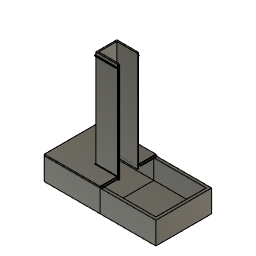
Tower+Base (Autodesk Fusion 360 design; units mm, degrees)
Autodesk Fusion 360 part; units mm, degrees
(part 1 of 2)
sketch "Sketch1" plane through (0, 0, 0) normal (0, 0, 1) x (1, 0, 0)
  line L0 (-38.1, 25.4) -> (469.9, 25.4)
  line L1 (469.9, 25.4) -> (469.9, -482.6)
  line L2 (469.9, -482.6) -> (-38.1, -482.6)
  line L3 (-38.1, -482.6) -> (-38.1, 25.4)
  dimension "d9" = 508
  dimension "d10" = 508
  constraint horizontal L0
  constraint vertical L1
  constraint horizontal L2
  constraint vertical L3
  measures "d9" distance of L0.start L0.end
  measures "d10" distance of L0.start L2.end
extrude "Extrude1" add sketch "Sketch1" along normal blind 203.2 makes body 1
sketch "Sketch2" plane through (0, 0, 203.2) normal (0, 0, 1) x (-1, 0, 0)
  line L0 (38.1, 482.6) -> (-469.9, 482.6)
  line L1 (-469.9, 482.6) -> (-469.9, -25.4)
  line L2 (-469.9, -25.4) -> (38.1, -25.4)
  line L3 (38.1, -25.4) -> (38.1, 482.6)
  line L4 (-469.9, 0) -> (12.7, 0)
  line L5 (12.7, 0) -> (12.7, 457.2)
  line L6 (12.7, 457.2) -> (-469.9, 457.2)
  line L7 (-469.9, 457.2) -> (-469.9, 0)
  dimension "d13" = 25.4
  dimension "d14" = 25.4
  dimension "d15" = 25.4
  constraint horizontal L4
  constraint vertical L5
  constraint horizontal L6
  constraint vertical L7
  constraint coincident L1 L4.start
  measures "d13" distance of L2 L4
  measures "d14" distance of L3 L5
  measures "d15" distance of L0 L6
extrude "Extrude2" cut sketch "Sketch2" against normal blind 177.8 contours L1 L4 L5 L6 L7 bodies 1
sketch "Sketch3" plane through (469.9, 0, 0) normal (1, 0, 0) x (0, 1, 0)
  line L0 (0, 203.2) -> (0, 25.4)
  line L1 (0, 25.4) -> (-457.2, 25.4)
  line L2 (-457.2, 25.4) -> (-457.2, 203.2)
  line L3 (-457.2, 203.2) -> (-482.6, 203.2)
  line L4 (-482.6, 203.2) -> (-482.6, 0)
  line L5 (-482.6, 0) -> (25.4, 0)
  line L6 (25.4, 0) -> (25.4, 203.2)
  line L7 (25.4, 203.2) -> (0, 203.2)
  line L8 (-457.2, 203.2) -> (-469.9, 203.2)
  line L9 (-469.9, 203.2) -> (-469.9, 12.7)
  line L10 (-469.9, 12.7) -> (-101.6, 12.7)
  line L11 (-101.6, 12.7) -> (12.7, 12.7)
  line L12 (12.7, 12.7) -> (12.7, 25.4)
  line L13 (0, 203.2) -> (12.7, 203.2)
  line L14 (12.7, 203.2) -> (12.7, 25.4)
  line L15 (0, 25.4) -> (0, 203.2)
  dimension "d20" = 12.7
  dimension "d21" = 12.7
  dimension "d22" = 12.7
  constraint horizontal L8
  constraint vertical L9
  constraint horizontal L10
  constraint coincident L2.end L3.start
  constraint horizontal L11
  constraint vertical L12
  constraint horizontal L13
  constraint vertical L14
  constraint vertical L15
  constraint coincident L0.start L7.end
  measures "d20" distance of L4 L9
  measures "d21" distance of L5 L11
  measures "d22" distance of L6 L14
extrude "Extrude3" add sketch "Sketch3" along normal blind 6.35 contours L0 L1 L2 L3 L7 L8 L9 L10 L11 L12 L13 L14 L15 bodies 1
move_body "Move1" bodies 1 to x (1, 0, 0) y (0, 1, 0) z (0, 0, 1) at (-317.5, 0, 0)
sketch "Sketch4" plane through (0, 0, 0) normal (0, 0, 1) x (1, 0, 0)
  line L0 (-127, 25.4) -> (381, 25.4)
  line L1 (381, 25.4) -> (381, -482.6)
  line L2 (381, -482.6) -> (-127, -482.6)
  line L3 (-127, -482.6) -> (-127, 25.4)
  dimension "d26" = 508
  dimension "d27" = 508
  constraint horizontal L0
  constraint vertical L1
  constraint horizontal L2
  constraint vertical L3
  measures "d26" distance of L0.start L0.end
  measures "d27" distance of L0.end L1.end
extrude "Extrude4" add sketch "Sketch4" along normal blind 203.2 separate body makes body 2
sketch "Sketch5" plane through (0, 0, 203.2) normal (0, 0, 1) x (-1, 0, 0)
  line L0 (127, 482.6) -> (-381, 482.6)
  line L1 (-381, 482.6) -> (-381, -25.4)
  line L2 (-381, -25.4) -> (127, -25.4)
  line L3 (127, -25.4) -> (127, 482.6)
  line L4 (127, 0) -> (-355.6, 0)
  line L5 (-355.6, 0) -> (-355.6, 457.2)
  line L6 (-355.6, 457.2) -> (127, 457.2)
  line L7 (127, 457.2) -> (127, 0)
  dimension "d30" = 25.4
  dimension "d31" = 25.4
  dimension "d32" = 25.4
  constraint horizontal L4
  constraint vertical L5
  constraint horizontal L6
  constraint vertical L7
  constraint coincident L3 L4.start
  measures "d30" distance of L2 L4
  measures "d31" distance of L1 L5
  measures "d32" distance of L0 L6
extrude "Extrude5" cut sketch "Sketch5" against normal blind 177.8 contours L3 L4 L5 L6 L7 bodies 2
sketch "Sketch6" plane through (-127, 0, 0) normal (-1, 0, 0) x (0, -1, 0)
  line L0 (457.2, 203.2) -> (457.2, 25.4)
  line L1 (457.2, 25.4) -> (0, 25.4)
  line L2 (0, 25.4) -> (0, 203.2)
  line L3 (0, 203.2) -> (-25.4, 203.2)
  line L4 (-25.4, 203.2) -> (-25.4, 0)
  line L5 (-25.4, 0) -> (482.6, 0)
  line L6 (482.6, 0) -> (482.6, 203.2)
  line L7 (482.6, 203.2) -> (457.2, 203.2)
  line L8 (0, 203.2) -> (-12.7, 203.2)
  line L9 (-12.7, 203.2) -> (-12.7, 12.7)
  line L10 (-12.7, 12.7) -> (0, 12.7)
  line L11 (0, 12.7) -> (469.9, 12.7)
  line L12 (469.9, 12.7) -> (469.9, 25.4)
  line L13 (457.2, 25.4) -> (457.2, 203.2)
  line L14 (457.2, 203.2) -> (469.9, 203.2)
  line L15 (469.9, 203.2) -> (469.9, 25.4)
  dimension "d35" = 12.7
  dimension "d36" = 12.7
  dimension "d37" = 12.7
  constraint horizontal L8
  constraint vertical L9
  constraint horizontal L10
  constraint coincident L2.end L3.start
  constraint horizontal L11
  constraint vertical L12
  constraint vertical L13
  constraint horizontal L14
  constraint vertical L15
  constraint coincident L0.start L7.end
  measures "d35" distance of L2 L9
  measures "d36" distance of L13 L15
  measures "d37" distance of L1 L11
extrude "Extrude6" cut sketch "Sketch6" against normal blind 6.35 contours L0 L1 L2 L3 L7 L8 L9 L10 L11 L12 L13 L14 L15 bodies 2
sketch "Sketch7" plane through (0, 0, 0) normal (0, 0, 1) x (1, 0, 0)
  line L0 (-457.2, 177.8) -> (50.8, 177.8)
  line L1 (50.8, 177.8) -> (50.8, -330.2)
  line L2 (50.8, -330.2) -> (-457.2, -330.2)
  line L3 (-457.2, -330.2) -> (-457.2, 177.8)
  line L4 (50.8, 25.4) -> (-152.4, 25.4)
  line L5 (-152.4, 25.4) -> (-152.4, -177.8)
  line L6 (-152.4, -177.8) -> (50.8, -177.8)
  line L7 (50.8, -177.8) -> (50.8, 25.4)
  dimension "d40" = 508
  dimension "d41" = 508
  dimension "d42" = 203.2
  dimension "d43" = 203.2
  dimension "d87" = 152.4
  constraint horizontal L0
  constraint vertical L1
  constraint horizontal L2
  constraint vertical L3
  constraint horizontal L4
  constraint vertical L5
  constraint horizontal L6
  constraint vertical L7
  constraint coincident L1 L4.start
  measures "d40" distance of L0.start L0.end
  measures "d41" distance of L0.start L2.end
  measures "d42" distance of L4.end L5.end
  measures "d43" distance of L4.start L4.end
  measures "d87" distance of L0 L4
extrude "Extrude7" add sketch "Sketch7" along normal blind 12.7 separate body contours L0 L1 L2 L3 L4 L5 L6 makes body 3
sketch "Sketch8" plane through (50.8, 0, 0) normal (1, 0, 0) x (0, 1, 0)
  line L0 (-330.2, 0) -> (-177.8, 0)
  line L1 (-177.8, 0) -> (-177.8, 12.7)
  line L2 (-177.8, 12.7) -> (-330.2, 12.7)
  line L3 (-330.2, 12.7) -> (-330.2, 0)
  line L4 (-330.2, 6.35) -> (-177.8, 6.35)
  line L5 (-177.8, 6.35) -> (-177.8, 0)
  line L6 (-177.8, 0) -> (-330.2, 0)
  line L7 (-330.2, 0) -> (-330.2, 6.35)
  dimension "d47" = 6.35
  constraint horizontal L4
  constraint vertical L5
  constraint horizontal L6
  constraint vertical L7
  constraint coincident L0.end L1.start
  constraint coincident L3 L4.start
  measures "d47" distance of L4.start L0.start
extrude "Extrude8" add sketch "Sketch8" along normal blind 12.7 contours L0 L1 L3 L4 L5 L6 L7 bodies 3
sketch "Sketch9" plane through (-152.4, 0, 0) normal (1, 0, 0) x (0, 1, 0)
  line L0 (-177.8, 0) -> (25.4, 0)
  line L1 (25.4, 0) -> (25.4, 12.7)
  line L2 (25.4, 12.7) -> (-177.8, 12.7)
  line L3 (-177.8, 12.7) -> (-177.8, 0)
  line L4 (-177.8, 0) -> (25.4, 0)
  line L5 (25.4, 0) -> (25.4, 6.35)
  line L6 (25.4, 6.35) -> (-177.8, 6.35)
  line L7 (-177.8, 6.35) -> (-177.8, 0)
  dimension "d51" = 6.35
  constraint horizontal L4
  constraint vertical L5
  constraint horizontal L6
  constraint vertical L7
  constraint coincident L1 L5.end
  constraint coincident L0.start L3.end
  measures "d51" distance of L0.start L6.end
extrude "Extrude9" add sketch "Sketch9" along normal blind 12.7 contours L0 L1 L3 L4 L5 L6 L7 bodies 3
sketch "Sketch10" plane through (50.8, 0, 0) normal (1, 0, 0) x (0, 1, 0)
  line L0 (25.4, 0) -> (177.8, 0)
  line L1 (177.8, 0) -> (177.8, 12.7)
  line L2 (177.8, 12.7) -> (25.4, 12.7)
  line L3 (25.4, 12.7) -> (25.4, 0)
  line L4 (25.4, 0) -> (177.8, 0)
  line L5 (177.8, 0) -> (177.8, 6.35)
  line L6 (177.8, 6.35) -> (25.4, 6.35)
  line L7 (25.4, 6.35) -> (25.4, 0)
  dimension "d54" = 6.35
  constraint horizontal L4
  constraint vertical L5
  constraint horizontal L6
  constraint vertical L7
  constraint coincident L1 L5.end
  constraint coincident L0.start L3.end
  measures "d54" distance of L0.start L6.end
extrude "Extrude10" add sketch "Sketch10" along normal blind 12.7 contours L0 L1 L3 L4 L5 L6 L7 bodies 3
sketch "Sketch11" plane through (0, -177.8, 0) normal (0, 1, 0) x (-1, 0, 0)
  line L0 (139.7, 6.35) -> (152.4, 6.35)
  line L1 (152.4, 6.35) -> (152.4, 12.7)
  line L2 (152.4, 12.7) -> (-50.8, 12.7)
  line L3 (-50.8, 12.7) -> (-50.8, 6.35)
  line L4 (-50.8, 6.35) -> (-63.5, 6.35)
  line L5 (-63.5, 6.35) -> (-63.5, 0)
  line L6 (-63.5, 0) -> (139.7, 0)
  line L7 (139.7, 0) -> (139.7, 6.35)
  line L8 (-50.8, 6.35) -> (139.7, 6.35)
  line L9 (139.7, 6.35) -> (139.7, 0)
  line L10 (139.7, 0) -> (-50.8, 0)
  line L11 (-50.8, 0) -> (-50.8, 6.35)
  constraint horizontal L8
  constraint vertical L9
  constraint horizontal L10
  constraint vertical L11
  constraint coincident L6.end L7.start
  constraint coincident L3.end L4.start
extrude "Extrude11" add sketch "Sketch11" along normal blind 12.7 contours L6 L7 L8 L9 L10 L11 bodies 3
sketch "Sketch12" plane through (0, 25.4, 0) normal (0, -1, 0) x (1, 0, 0)
  line L0 (-152.4, 6.35) -> (-139.7, 6.35)
  line L1 (-139.7, 6.35) -> (-139.7, 0)
  line L2 (-139.7, 0) -> (63.5, 0)
  line L3 (63.5, 0) -> (63.5, 6.35)
  line L4 (63.5, 6.35) -> (50.8, 6.35)
  line L5 (50.8, 6.35) -> (50.8, 12.7)
  line L6 (50.8, 12.7) -> (-152.4, 12.7)
  line L7 (-152.4, 12.7) -> (-152.4, 6.35)
  line L8 (-139.7, 0) -> (50.8, 0)
  line L9 (50.8, 0) -> (50.8, 6.35)
  line L10 (50.8, 6.35) -> (-139.7, 6.35)
  line L11 (-139.7, 6.35) -> (-139.7, 0)
  constraint horizontal L8
  constraint vertical L9
  constraint horizontal L10
  constraint vertical L11
  constraint coincident L4.end L5.start
  constraint coincident L1.end L2.start
extrude "Extrude12" add sketch "Sketch12" along normal blind 12.7 contours L1 L2 L8 L9 L10 L11 bodies 3
sketch "Sketch13" plane through (0, 0, 0) normal (0, 0, 1) x (1, 0, 0)
  line L0 (-152.4, 177.8) -> (355.6, 177.8)
  line L1 (355.6, 177.8) -> (355.6, -330.2)
  line L2 (355.6, -330.2) -> (-152.4, -330.2)
  line L3 (-152.4, -330.2) -> (-152.4, 177.8)
  line L4 (-152.4, 25.4) -> (50.8, 25.4)
  line L5 (50.8, 25.4) -> (50.8, -177.8)
  line L6 (50.8, -177.8) -> (-152.4, -177.8)
  line L7 (-152.4, -177.8) -> (-152.4, 25.4)
  dimension "d61" = 508
  dimension "d62" = 508
  dimension "d63" = 203.2
  dimension "d64" = 203.2
  dimension "d88" = 152.4
  constraint horizontal L0
  constraint vertical L1
  constraint horizontal L2
  constraint vertical L3
  constraint horizontal L4
  constraint vertical L5
  constraint horizontal L6
  constraint vertical L7
  constraint coincident L3 L4.start
  measures "d61" distance of L0.start L0.end
  measures "d62" distance of L0.end L1.end
  measures "d63" distance of L4.start L4.end
  measures "d64" distance of L4.end L5.end
  measures "d88" distance of L0 L4
extrude "Extrude13" add sketch "Sketch13" along normal blind 12.7 separate body contours L0 L1 L2 L3 L4 L5 L6 makes body 4
sketch "Sketch14" plane through (-152.4, 0, 0) normal (-1, 0, 0) x (0, -1, 0)
  line L0 (-177.8, 0) -> (-25.4, 0)
  line L1 (-25.4, 0) -> (-25.4, 12.7)
  line L2 (-25.4, 12.7) -> (-177.8, 12.7)
  line L3 (-177.8, 12.7) -> (-177.8, 0)
  line L4 (-177.8, 0) -> (-25.4, 0)
  line L5 (-25.4, 0) -> (-25.4, 6.35)
  line L6 (-25.4, 6.35) -> (-177.8, 6.35)
  line L7 (-177.8, 6.35) -> (-177.8, 0)
  dimension "d67" = 6.35
  constraint horizontal L4
  constraint vertical L5
  constraint horizontal L6
  constraint vertical L7
  constraint coincident L1 L5.end
  constraint coincident L0.start L3.end
  measures "d67" distance of L0.start L6.end
extrude "Extrude14" cut sketch "Sketch14" against normal blind 12.7 contours L0 L1 L3 L4 L5 L6 L7 bodies 4
sketch "Sketch15" plane through (-152.4, 0, 0) normal (-1, 0, 0) x (0, -1, 0)
  line L0 (177.8, 0) -> (330.2, 0)
  line L1 (330.2, 0) -> (330.2, 12.7)
  line L2 (330.2, 12.7) -> (177.8, 12.7)
  line L3 (177.8, 12.7) -> (177.8, 0)
  line L4 (177.8, 0) -> (330.2, 0)
  line L5 (330.2, 0) -> (330.2, 6.35)
  line L6 (330.2, 6.35) -> (177.8, 6.35)
  line L7 (177.8, 6.35) -> (177.8, 0)
  dimension "d70" = 6.35
  constraint horizontal L4
  constraint vertical L5
  constraint horizontal L6
  constraint vertical L7
  constraint coincident L1 L5.end
  constraint coincident L0.start L3.end
  measures "d70" distance of L0.start L6.end
extrude "Extrude15" cut sketch "Sketch15" against normal blind 12.7 contours L0 L1 L3 L4 L5 L6 L7 bodies 4
sketch "Sketch16" plane through (50.8, 0, 0) normal (-1, 0, 0) x (0, -1, 0)
  line L0 (-25.4, 0) -> (177.8, 0)
  line L1 (177.8, 0) -> (177.8, 12.7)
  line L2 (177.8, 12.7) -> (-25.4, 12.7)
  line L3 (-25.4, 12.7) -> (-25.4, 0)
  line L4 (-25.4, 0) -> (177.8, 0)
  line L5 (177.8, 0) -> (177.8, 12.7)
  line L6 (177.8, 12.7) -> (-25.4, 12.7)
  line L7 (-25.4, 12.7) -> (-25.4, 0)
  dimension "d73" = 12.7
  constraint horizontal L4
  constraint vertical L5
  constraint horizontal L6
  constraint vertical L7
  constraint coincident L1 L2.start
  constraint coincident L0.start L3.end
  measures "d73" distance of L0.start L2.end
extrude "Extrude16" add sketch "Sketch16" along normal blind 12.7 bodies 4
sketch "Sketch17" plane through (0, 25.4, 0) normal (0, -1, 0) x (1, 0, 0)
  line L0 (38.1, 0) -> (38.1, 12.7)
  line L1 (-152.4, 12.7) -> (-152.4, 6.35)
  line L2 (-152.4, 6.35) -> (-139.7, 6.35)
  line L3 (-139.7, 6.35) -> (-139.7, 0)
  line L4 (-139.7, 0) -> (38.1, 0)
  line L5 (-139.7, 0) -> (38.1, 0)
  line L6 (38.1, 0) -> (38.1, 12.7)
  line L7 (38.1, 12.7) -> (-139.7, 12.7)
  line L8 (-139.7, 12.7) -> (-139.7, 0)
  line L9 (38.1, 12.7) -> (-152.4, 12.7)
  constraint horizontal L5
  constraint vertical L6
  constraint horizontal L7
  constraint vertical L8
  constraint coincident L0.end L6.end
  constraint coincident L3.end L4.start
extrude "Extrude17" add sketch "Sketch17" along normal blind 12.7 contours L0 L3 L4 L5 L6 L7 L8 L9 bodies 4
sketch "Sketch18" plane through (0, -177.8, 0) normal (0, 1, 0) x (-1, 0, 0)
  line L0 (152.4, 12.7) -> (-38.1, 12.7)
  line L1 (-38.1, 12.7) -> (-38.1, 0)
  line L2 (-38.1, 0) -> (139.7, 0)
  line L3 (139.7, 0) -> (139.7, 6.35)
  line L4 (139.7, 6.35) -> (152.4, 6.35)
  line L5 (152.4, 6.35) -> (152.4, 12.7)
  line L6 (-38.1, 0) -> (139.7, 0)
  line L7 (139.7, 0) -> (139.7, 6.35)
  line L8 (139.7, 6.35) -> (-38.1, 6.35)
  line L9 (-38.1, 6.35) -> (-38.1, 0)
  constraint horizontal L6
  constraint vertical L7
  constraint horizontal L8
  constraint vertical L9
  constraint coincident L3.end L4.start
  constraint coincident L1.end L2.start
extrude "Extrude18" add sketch "Sketch18" along normal blind 12.7 contours L1 L2 L3 L6 L7 L8 L9 bodies 4
sketch "Sketch19" plane through (-139.7, 0, 0) normal (-1, 0, 0) x (0, -1, 0)
  line L0 (-177.8, 6.35) -> (-177.8, 0)
  line L1 (-177.8, 0) -> (-12.7, 0)
  line L2 (-12.7, 0) -> (-12.7, 12.7)
  line L3 (-12.7, 12.7) -> (-25.4, 12.7)
  line L4 (-25.4, 6.35) -> (-177.8, 6.35)
  line L5 (-25.4, 12.7) -> (-12.7, 12.7)
  line L6 (-12.7, 12.7) -> (-12.7, 0)
  line L7 (-12.7, 0) -> (-25.4, 0)
  line L8 (-25.4, 0) -> (-25.4, 12.7)
  line L9 (-25.4, 12.7) -> (-25.4, 6.35)
  constraint horizontal L5
  constraint vertical L6
  constraint horizontal L7
  constraint vertical L8
  constraint coincident L1.end L2.start
  constraint coincident L3.end L5.start
sketch "Sketch20" plane through (-139.7, 0, 0) normal (-1, 0, 0) x (0, -1, 0)
  line L0 (165.1, 0) -> (330.2, 0)
  line L1 (330.2, 0) -> (330.2, 6.35)
  line L2 (330.2, 6.35) -> (177.8, 6.35)
  line L3 (177.8, 6.35) -> (165.1, 6.35)
  line L4 (165.1, 6.35) -> (165.1, 0)
  line L5 (165.1, 6.35) -> (177.8, 6.35)
  line L6 (177.8, 6.35) -> (177.8, 0)
  line L7 (177.8, 0) -> (165.1, 0)
  line L8 (165.1, 0) -> (165.1, 6.35)
  constraint horizontal L5
  constraint vertical L6
  constraint horizontal L7
  constraint vertical L8
  constraint coincident L0 L6.end
  constraint coincident L3.end L4.start
extrude "Extrude20" add sketch "Sketch20" along normal blind 12.7 separate body contours L0 L3 L4 L5 L6 L7 L8 makes body 5
sketch "Sketch21" plane through (-139.7, 0, 0) normal (-1, 0, 0) x (0, -1, 0)
  line L0 (-177.8, 6.35) -> (-177.8, 0)
  line L1 (-177.8, 0) -> (-12.7, 0)
  line L2 (-12.7, 0) -> (-12.7, 12.7)
  line L3 (-12.7, 12.7) -> (-25.4, 12.7)
  line L4 (-25.4, 6.35) -> (-177.8, 6.35)
  line L5 (-25.4, 12.7) -> (-12.7, 12.7)
  line L6 (-12.7, 12.7) -> (-12.7, 0)
  line L7 (-12.7, 0) -> (-25.4, 0)
  line L8 (-25.4, 0) -> (-25.4, 12.7)
  line L9 (-25.4, 12.7) -> (-25.4, 6.35)
  constraint horizontal L5
  constraint vertical L6
  constraint horizontal L7
  constraint vertical L8
  constraint coincident L1.end L2.start
  constraint coincident L3.end L5.start
extrude "Extrude21" add sketch "Sketch21" along normal blind 12.7 separate body contours L1 L2 L3 L5 L6 L7 L8 L9 makes body 6
combine "Combine1" operation add target body 6 tool bodies 4 5
sketch "Sketch22" plane through (0, 0, 0) normal (0, 0, 1) x (1, 0, 0)
sketch "Sketch23" plane through (0, 0, 0) normal (0, 0, 1) x (1, 0, 0)
sketch "Sketch24" plane through (0, 314.0699, 0) normal (0, 1, 0) x (-1, 0, 0)
  line L0 (-261.6067, 0) -> (-198.1067, 0)
  line L1 (-198.1067, 0) -> (-198.1067, 152.4)
  line L2 (-198.1067, 152.4) -> (-261.6067, 152.4)
  line L3 (-261.6067, 152.4) -> (-261.6067, 0)
  line L4 (-261.6067, 25.4) -> (-198.1067, 25.4)
  line L5 (-198.1067, 25.4) -> (-198.1067, 38.1)
  line L6 (-198.1067, 38.1) -> (-261.6067, 38.1)
  line L7 (-261.6067, 38.1) -> (-261.6067, 25.4)
  dimension "d96" = 25.4
  dimension "d97" = 12.7
  constraint horizontal L4
  constraint vertical L5
  constraint horizontal L6
  constraint vertical L7
  constraint coincident L1 L5.end
  constraint coincident L3 L4.start
  measures "d96" distance of L0 L4
  measures "d97" distance of L4.start L6.end
sketch "Sketch25" plane through (0, 314.0699, 0) normal (0, 1, 0) x (-1, 0, 0)
  line L0 (-261.6067, 38.1) -> (-198.1067, 38.1)
  line L1 (-198.1067, 38.1) -> (-198.1067, 152.4)
  line L2 (-198.1067, 152.4) -> (-261.6067, 152.4)
  line L3 (-261.6067, 152.4) -> (-261.6067, 38.1)
  line L4 (-261.6067, 127) -> (-198.1067, 127)
  line L5 (-198.1067, 127) -> (-198.1067, 114.3)
  line L6 (-198.1067, 114.3) -> (-261.6067, 114.3)
  line L7 (-261.6067, 114.3) -> (-261.6067, 127)
  dimension "d100" = 25.4
  dimension "d101" = 12.7
  constraint horizontal L4
  constraint vertical L5
  constraint horizontal L6
  constraint vertical L7
  constraint coincident L1 L5.end
  constraint coincident L3 L4.start
  measures "d100" distance of L2 L4
  measures "d101" distance of L4.end L5.end
sketch "Sketch26" plane through (0, 187.0699, 0) normal (0, -1, 0) x (1, 0, 0)
  line L0 (198.1067, 0) -> (261.6067, 0)
  line L1 (261.6067, 0) -> (261.6067, 152.4)
  line L2 (261.6067, 152.4) -> (198.1067, 152.4)
  line L3 (198.1067, 152.4) -> (198.1067, 0)
  line L4 (198.1067, 127) -> (261.6067, 127)
  line L5 (261.6067, 127) -> (261.6067, 114.3)
  line L6 (261.6067, 114.3) -> (198.1067, 114.3)
  line L7 (198.1067, 114.3) -> (198.1067, 127)
  dimension "d104" = 12.7
  dimension "d105" = 25.4
  constraint horizontal L4
  constraint vertical L5
  constraint horizontal L6
  constraint vertical L7
  constraint coincident L1 L5.end
  constraint coincident L3 L4.start
  measures "d104" distance of L4.start L6.end
  measures "d105" distance of L2 L4
sketch "Sketch27" plane through (0, 187.0699, 0) normal (0, -1, 0) x (1, 0, 0)
  line L0 (261.6067, 114.3) -> (198.1067, 114.3)
  line L1 (198.1067, 114.3) -> (198.1067, 0)
  line L2 (198.1067, 0) -> (261.6067, 0)
  line L3 (261.6067, 0) -> (261.6067, 114.3)
  line L4 (198.1067, 25.4) -> (261.6067, 25.4)
  line L5 (261.6067, 25.4) -> (261.6067, 38.1)
  line L6 (261.6067, 38.1) -> (198.1067, 38.1)
  line L7 (198.1067, 38.1) -> (198.1067, 25.4)
  dimension "d108" = 25.4
  dimension "d109" = 12.7
  constraint horizontal L4
  constraint vertical L5
  constraint horizontal L6
  constraint vertical L7
  constraint coincident L3 L5.end
  constraint coincident L1 L4.start
  measures "d108" distance of L2 L4
  measures "d109" distance of L4 L6
sketch "Sketch28" plane through (198.1067, 0, 0) normal (-1, 0, 0) x (0, -1, 0)
  line L0 (-314.0699, 127) -> (-326.7699, 127)
  line L1 (-326.7699, 127) -> (-326.7699, 114.3)
  line L2 (-326.7699, 114.3) -> (-314.0699, 114.3)
  line L3 (-326.7699, 127) -> (-174.3699, 127)
  line L4 (-174.3699, 127) -> (-174.3699, 114.3)
  line L5 (-174.3699, 114.3) -> (-326.7699, 114.3)
  line L6 (-326.7699, 114.3) -> (-326.7699, 127)
  line L7 (-314.0699, 114.3) -> (-314.0699, 127)
  constraint horizontal L3
  constraint vertical L4
  constraint horizontal L5
  constraint vertical L6
  constraint coincident L0.end L1.start
sketch "Sketch29" plane through (198.1067, 0, 0) normal (-1, 0, 0) x (0, -1, 0)
  line L0 (-314.0699, 38.1) -> (-326.7699, 38.1)
  line L1 (-326.7699, 38.1) -> (-326.7699, 25.4)
  line L2 (-326.7699, 25.4) -> (-314.0699, 25.4)
  line L3 (-326.7699, 38.1) -> (-174.3699, 38.1)
  line L4 (-174.3699, 38.1) -> (-174.3699, 25.4)
  line L5 (-174.3699, 25.4) -> (-326.7699, 25.4)
  line L6 (-326.7699, 25.4) -> (-326.7699, 38.1)
  line L7 (-314.0699, 25.4) -> (-314.0699, 38.1)
  constraint horizontal L3
  constraint vertical L4
  constraint horizontal L5
  constraint vertical L6
  constraint coincident L0.end L1.start
sketch "Sketch30" plane through (299.7067, 0, 0) normal (-1, 0, 0) x (0, -1, 0)
  line L0 (-301.3699, 0) -> (-288.6699, 0)
  line L1 (-288.6699, 0) -> (-288.6699, 152.4)
  line L2 (-288.6699, 152.4) -> (-301.3699, 152.4)
  line L3 (-301.3699, 152.4) -> (-301.3699, 127)
  line L4 (-301.3699, 127) -> (-314.0699, 127)
  line L5 (-314.0699, 127) -> (-314.0699, 114.3)
  line L6 (-314.0699, 114.3) -> (-301.3699, 114.3)
  line L7 (-301.3699, 114.3) -> (-301.3699, 38.1)
  line L8 (-301.3699, 38.1) -> (-314.0699, 38.1)
  line L9 (-314.0699, 38.1) -> (-314.0699, 25.4)
  line L10 (-314.0699, 25.4) -> (-301.3699, 25.4)
  line L11 (-301.3699, 25.4) -> (-301.3699, 0)
  line L12 (-288.6699, 0) -> (-295.0199, 0)
  line L13 (-295.0199, 0) -> (-295.0199, 152.4)
  line L14 (-295.0199, 152.4) -> (-288.6699, 152.4)
  line L15 (-288.6699, 152.4) -> (-288.6699, 0)
  constraint horizontal L12
  constraint vertical L13
  constraint horizontal L14
  constraint vertical L15
  constraint midpoint L2 L13.end
  constraint coincident L0.end L1.start
sketch "Sketch31" plane through (287.0067, 0, 0) normal (-1, 0, 0) x (0, -1, 0)
  line L0 (-288.6699, 152.4) -> (-295.0199, 152.4)
  line L1 (-295.0199, 152.4) -> (-295.0199, 0)
  line L2 (-295.0199, 0) -> (-288.6699, 0)
  line L3 (-288.6699, 0) -> (-288.6699, 152.4)
  line L4 (-295.0199, 152.4) -> (-288.6699, 152.4)
  line L5 (-288.6699, 152.4) -> (-288.6699, 139.7)
  line L6 (-288.6699, 139.7) -> (-295.0199, 139.7)
  line L7 (-295.0199, 139.7) -> (-295.0199, 152.4)
  dimension "d120" = 12.7
  constraint horizontal L4
  constraint vertical L5
  constraint horizontal L6
  constraint vertical L7
  constraint coincident L3 L5.end
  constraint coincident L0.end L1.start
  measures "d120" distance of L0.end L6.end
sketch "Sketch32" plane through (299.7067, 0, 0) normal (-1, 0, 0) x (0, -1, 0)
  line L0 (-187.0699, 0) -> (-174.3699, 0)
  line L1 (-174.3699, 0) -> (-174.3699, 25.4)
  line L2 (-174.3699, 25.4) -> (-161.6699, 25.4)
  line L3 (-161.6699, 25.4) -> (-161.6699, 38.1)
  line L4 (-161.6699, 38.1) -> (-174.3699, 38.1)
  line L5 (-174.3699, 38.1) -> (-174.3699, 114.3)
  line L6 (-174.3699, 114.3) -> (-161.6699, 114.3)
  line L7 (-161.6699, 114.3) -> (-161.6699, 127)
  line L8 (-161.6699, 127) -> (-174.3699, 127)
  line L9 (-174.3699, 127) -> (-174.3699, 152.4)
  line L10 (-174.3699, 152.4) -> (-187.0699, 152.4)
  line L11 (-187.0699, 152.4) -> (-187.0699, 0)
  line L12 (-187.0699, 152.4) -> (-180.7199, 152.4)
  line L13 (-180.7199, 152.4) -> (-180.7199, 0)
  line L14 (-180.7199, 0) -> (-187.0699, 0)
  line L15 (-187.0699, 0) -> (-187.0699, 152.4)
  constraint horizontal L12
  constraint vertical L13
  constraint horizontal L14
  constraint vertical L15
  constraint midpoint L0 L13.end
  constraint coincident L10.end L11.start
sketch "Sketch33" plane through (287.0067, 0, 0) normal (-1, 0, 0) x (0, -1, 0)
  line L0 (-187.0699, 0) -> (-180.7199, 0)
  line L1 (-180.7199, 0) -> (-180.7199, 152.4)
  line L2 (-180.7199, 152.4) -> (-187.0699, 152.4)
  line L3 (-187.0699, 152.4) -> (-187.0699, 0)
  line L4 (-187.0699, 152.4) -> (-180.7199, 152.4)
  line L5 (-180.7199, 152.4) -> (-180.7199, 139.7)
  line L6 (-180.7199, 139.7) -> (-187.0699, 139.7)
  line L7 (-187.0699, 139.7) -> (-187.0699, 152.4)
  dimension "d125" = 12.7
  constraint horizontal L4
  constraint vertical L5
  constraint horizontal L6
  constraint vertical L7
  constraint coincident L1 L5.end
  constraint coincident L2.end L3.start
  measures "d125" distance of L1.end L5.end
sketch "Sketch34" plane through (261.6067, 0, 0) normal (1, 0, 0) x (0, 1, 0)
  line L0 (187.0699, 127) -> (174.3699, 127)
  line L1 (174.3699, 127) -> (174.3699, 114.3)
  line L2 (174.3699, 114.3) -> (187.0699, 114.3)
  line L3 (199.7699, 0) -> (187.0699, 0)
  line L4 (187.0699, 0) -> (187.0699, 139.7)
  line L5 (187.0699, 139.7) -> (199.7699, 139.7)
  line L6 (199.7699, 139.7) -> (199.7699, 0)
  line L7 (187.0699, 114.3) -> (187.0699, 127)
  constraint horizontal L3
  constraint vertical L4
  constraint horizontal L5
  constraint vertical L6
sketch "Sketch35" plane through (261.6067, 0, 0) normal (1, 0, 0) x (0, 1, 0)
  line L0 (314.0699, 114.3) -> (326.7699, 114.3)
  line L1 (326.7699, 114.3) -> (326.7699, 127)
  line L2 (326.7699, 127) -> (314.0699, 127)
  line L3 (301.3699, 0) -> (314.0699, 0)
  line L4 (314.0699, 0) -> (314.0699, 139.7)
  line L5 (314.0699, 139.7) -> (301.3699, 139.7)
  line L6 (301.3699, 139.7) -> (301.3699, 0)
  line L7 (314.0699, 127) -> (314.0699, 114.3)
  constraint horizontal L3
  constraint vertical L4
  constraint horizontal L5
  constraint vertical L6
move_body "Move3" bodies 6 to x (1, 0, 0) y (0, 1, 0) z (0, 0, 1) at (0, 152.4, 0)
move_body "Move4" bodies 3 to x (1, 0, 0) y (0, 1, 0) z (0, 0, 1) at (0, 127, 0)
move_body "Move5" bodies 1 to x (1, 0, 0) y (0, 1, 0) z (0, 0, 1) at (-25.4, 0, 0)
move_body "Move6" bodies 3 to x (1, 0, 0) y (0, 1, 0) z (0, 0, 1) at (63.5, -292.1, 152.4)
move_body "Move7" bodies 6 to x (1, 0, 0) y (0, 1, 0) z (0, 0, 1) at (25.4, -330.2, 152.4)
move_body "Move8" bodies 3 to x (1, 0, 0) y (0, 1, 0) z (0, 0, 1) at (12.7, -12.7, 0)
move_body "Move11" bodies 1 to x (1, 0, 0) y (0, 1, 0) z (0, 0, 1) at (-88.9, 0, 0)
move_body "Move12" bodies 3 to x (1, 0, 0) y (0, 1, 0) z (0, 0, 1) at (-88.9, 0, 0)
move_body "Move13" bodies 1 to x (1, 0, 0) y (0, 1, 0) z (0, 0, 1) at (-101.6, 0, 0)
move_body "Move14" bodies 3 to x (1, 0, 0) y (0, 1, 0) z (0, 0, 1) at (-101.6, 0, 0)
sketch "Sketch36" plane through (0, 0, 0) normal (0, 0, 1) x (1, 0, 0)
  line L0 (-203.2, 304.8) -> (-6.35, 304.8)
  line L1 (-6.35, 304.8) -> (-6.35, 114.3)
  line L2 (-6.35, 114.3) -> (-203.2, 114.3)
  line L3 (-203.2, 114.3) -> (-203.2, 304.8)
  line L4 (-6.35, 292.1) -> (-190.5, 292.1)
  line L5 (-190.5, 292.1) -> (-190.5, 127)
  line L6 (-190.5, 127) -> (-6.35, 127)
  line L7 (-6.35, 127) -> (-6.35, 292.1)
  dimension "d136" = 196.85
  dimension "d137" = 190.5
  dimension "d138" = 12.7
  dimension "d139" = 12.7
  dimension "d140" = 12.7
  constraint horizontal L0
  constraint vertical L1
  constraint horizontal L2
  constraint vertical L3
  constraint horizontal L4
  constraint vertical L5
  constraint horizontal L6
  constraint vertical L7
  constraint coincident L1 L4.start
  measures "d136" distance of L0.start L0.end
  measures "d137" distance of L0.start L2.end
  measures "d138" distance of L3 L5
  measures "d139" distance of L2 L6
  measures "d140" distance of L0 L4
extrude "Extrude36" add sketch "Sketch36" along normal blind 914.4 separate body contours L0 L1 L2 L3 L4 L5 L6 makes body 7
sketch "Sketch37" plane through (0, 304.8, 0) normal (0, 1, 0) x (-1, 0, 0)
  line L0 (6.35, 0) -> (203.2, 0)
  line L1 (203.2, 0) -> (203.2, 914.4)
  line L2 (203.2, 914.4) -> (6.35, 914.4)
  line L3 (6.35, 914.4) -> (6.35, 0)
  line L4 (6.35, 31.75) -> (203.2, 31.75)
  line L5 (203.2, 31.75) -> (203.2, 25.4)
  line L6 (203.2, 25.4) -> (6.35, 25.4)
  line L7 (6.35, 25.4) -> (6.35, 31.75)
  dimension "d143" = 25.4
  dimension "d146" = 6.35
  constraint horizontal L4
  constraint vertical L5
  constraint horizontal L6
  constraint vertical L7
  constraint coincident L1 L5.end
  constraint coincident L3 L4.start
  measures "d143" distance of L0 L6
  measures "d146" distance of L4.start L6.end
extrude "Extrude37" add sketch "Sketch37" along normal blind 6.35 contours L1 L3 L4 L5 L6 L7 bodies 7
sketch "Sketch38" plane through (0, 304.8, 0) normal (0, 1, 0) x (-1, 0, 0)
  line L0 (6.35, 31.75) -> (203.2, 31.75)
  line L1 (203.2, 31.75) -> (203.2, 914.4)
  line L2 (203.2, 914.4) -> (6.35, 914.4)
  line L3 (6.35, 914.4) -> (6.35, 31.75)
  line L4 (6.35, 889) -> (203.2, 889)
  line L5 (203.2, 889) -> (203.2, 882.65)
  line L6 (203.2, 882.65) -> (6.35, 882.65)
  line L7 (6.35, 882.65) -> (6.35, 889)
  dimension "d149" = 25.4
  dimension "d150" = 6.35
  constraint horizontal L4
  constraint vertical L5
  constraint horizontal L6
  constraint vertical L7
  constraint coincident L1 L5.end
  constraint coincident L3 L4.start
  measures "d149" distance of L2 L4
  measures "d150" distance of L4.start L6.end
extrude "Extrude38" add sketch "Sketch38" along normal blind 6.35 contours L1 L3 L4 L5 L6 L7 bodies 7
sketch "Sketch39" plane through (0, 114.3, 0) normal (0, -1, 0) x (1, 0, 0)
  line L0 (-203.2, 0) -> (-6.35, 0)
  line L1 (-6.35, 0) -> (-6.35, 914.4)
  line L2 (-6.35, 914.4) -> (-203.2, 914.4)
  line L3 (-203.2, 914.4) -> (-203.2, 0)
  line L4 (-203.2, 889) -> (-6.35, 889)
  line L5 (-6.35, 889) -> (-6.35, 882.65)
  line L6 (-6.35, 882.65) -> (-203.2, 882.65)
  line L7 (-203.2, 882.65) -> (-203.2, 889)
  dimension "d153" = 25.4
  dimension "d154" = 6.35
  constraint horizontal L4
  constraint vertical L5
  constraint horizontal L6
  constraint vertical L7
  constraint coincident L1 L5.end
  constraint coincident L3 L4.start
  measures "d153" distance of L2 L4
  measures "d154" distance of L4.start L6.end
extrude "Extrude39" add sketch "Sketch39" along normal blind 6.35 contours L1 L3 L4 L5 L6 L7 bodies 7
sketch "Sketch40" plane through (0, 114.3, 0) normal (0, -1, 0) x (1, 0, 0)
  line L0 (-6.35, 882.65) -> (-203.2, 882.65)
  line L1 (-203.2, 882.65) -> (-203.2, 0)
  line L2 (-203.2, 0) -> (-6.35, 0)
  line L3 (-6.35, 0) -> (-6.35, 882.65)
  line L4 (-203.2, 31.75) -> (-6.35, 31.75)
  line L5 (-6.35, 31.75) -> (-6.35, 25.4)
  line L6 (-6.35, 25.4) -> (-203.2, 25.4)
  line L7 (-203.2, 25.4) -> (-203.2, 31.75)
  dimension "d157" = 25.4
  dimension "d158" = 6.35
  constraint horizontal L4
  constraint vertical L5
  constraint horizontal L6
  constraint vertical L7
  constraint coincident L3 L5.end
  constraint coincident L1 L4.start
  measures "d157" distance of L2 L6
  measures "d158" distance of L4.start L6.end
extrude "Extrude40" add sketch "Sketch40" along normal blind 6.35 contours L1 L3 L4 L5 L6 L7 bodies 7
sketch "Sketch41" plane through (-203.2, 0, 0) normal (-1, 0, 0) x (0, -1, 0)
  line L0 (-304.8, 0) -> (-114.3, 0)
  line L1 (-114.3, 0) -> (-114.3, 25.4)
  line L2 (-114.3, 25.4) -> (-107.95, 25.4)
  line L3 (-107.95, 25.4) -> (-107.95, 31.75)
  line L4 (-107.95, 31.75) -> (-114.3, 31.75)
  line L5 (-114.3, 31.75) -> (-114.3, 882.65)
  line L6 (-114.3, 882.65) -> (-107.95, 882.65)
  line L7 (-107.95, 882.65) -> (-107.95, 889)
  line L8 (-107.95, 889) -> (-114.3, 889)
  line L9 (-114.3, 889) -> (-114.3, 914.4)
  line L10 (-114.3, 914.4) -> (-304.8, 914.4)
  line L11 (-304.8, 914.4) -> (-304.8, 889)
  line L12 (-304.8, 889) -> (-311.15, 889)
  line L13 (-311.15, 889) -> (-311.15, 882.65)
  line L14 (-311.15, 882.65) -> (-304.8, 882.65)
  line L15 (-304.8, 882.65) -> (-304.8, 31.75)
  line L16 (-304.8, 31.75) -> (-311.15, 31.75)
  line L17 (-311.15, 31.75) -> (-311.15, 25.4)
  line L18 (-311.15, 25.4) -> (-304.8, 25.4)
  line L19 (-304.8, 25.4) -> (-304.8, 0)
  line L20 (-311.15, 889) -> (-107.95, 889)
  line L21 (-107.95, 889) -> (-107.95, 882.65)
  line L22 (-107.95, 882.65) -> (-311.15, 882.65)
  line L23 (-311.15, 882.65) -> (-311.15, 889)
  constraint horizontal L20
  constraint vertical L21
  constraint horizontal L22
  constraint vertical L23
  constraint coincident L6.end L7.start
  constraint coincident L12.end L13.start
extrude "Extrude41" add sketch "Sketch41" along normal blind 6.35 contours L6 L7 L8 L12 L13 L14 L20 L21 L22 L23 bodies 7
sketch "Sketch42" plane through (-203.2, 0, 0) normal (-1, 0, 0) x (0, -1, 0)
  line L0 (-114.3, 882.65) -> (-304.8, 882.65)
  line L1 (-304.8, 882.65) -> (-304.8, 31.75)
  line L2 (-304.8, 31.75) -> (-311.15, 31.75)
  line L3 (-311.15, 31.75) -> (-311.15, 25.4)
  line L4 (-311.15, 25.4) -> (-304.8, 25.4)
  line L5 (-304.8, 25.4) -> (-304.8, 0)
  line L6 (-304.8, 0) -> (-114.3, 0)
  line L7 (-114.3, 0) -> (-114.3, 25.4)
  line L8 (-114.3, 25.4) -> (-107.95, 25.4)
  line L9 (-107.95, 25.4) -> (-107.95, 31.75)
  line L10 (-107.95, 31.75) -> (-114.3, 31.75)
  line L11 (-114.3, 31.75) -> (-114.3, 882.65)
  line L12 (-311.15, 31.75) -> (-107.95, 31.75)
  line L13 (-107.95, 31.75) -> (-107.95, 25.4)
  line L14 (-107.95, 25.4) -> (-311.15, 25.4)
  line L15 (-311.15, 25.4) -> (-311.15, 31.75)
  constraint horizontal L12
  constraint vertical L13
  constraint horizontal L14
  constraint vertical L15
  constraint coincident L8.end L9.start
  constraint coincident L2.end L3.start
extrude "Extrude42" add sketch "Sketch42" along normal blind 6.35 contours L2 L3 L4 L8 L9 L10 L12 L13 L14 L15 bodies 7
sketch "Sketch43" plane through (-6.35, 0, 0) normal (1, 0, 0) x (0, 1, 0)
  line L0 (114.3, 0) -> (127, 0)
  line L1 (127, 0) -> (127, 914.4)
  line L2 (127, 914.4) -> (114.3, 914.4)
  line L3 (114.3, 914.4) -> (114.3, 889)
  line L4 (114.3, 889) -> (107.95, 889)
  line L5 (107.95, 889) -> (107.95, 882.65)
  line L6 (107.95, 882.65) -> (114.3, 882.65)
  line L7 (114.3, 882.65) -> (114.3, 31.75)
  line L8 (114.3, 31.75) -> (107.95, 31.75)
  line L9 (107.95, 31.75) -> (107.95, 25.4)
  line L10 (107.95, 25.4) -> (114.3, 25.4)
  line L11 (114.3, 25.4) -> (114.3, 0)
  line L12 (127, 914.4) -> (120.65, 914.4)
  line L13 (120.65, 914.4) -> (120.65, 0)
  line L14 (120.65, 0) -> (127, 0)
  line L15 (127, 0) -> (127, 914.4)
  line L16 (120.65, 914.4) -> (127, 914.4)
  line L17 (127, 914.4) -> (127, 908.05)
  line L18 (127, 908.05) -> (120.65, 908.05)
  line L19 (120.65, 908.05) -> (120.65, 914.4)
  dimension "d167" = 6.35
  dimension "d168" = 6.35
  constraint horizontal L12
  constraint vertical L13
  constraint horizontal L14
  constraint vertical L15
  constraint coincident L0 L13.end
  constraint coincident L1.end L2.start
  constraint horizontal L16
  constraint vertical L17
  constraint horizontal L18
  constraint vertical L19
  constraint coincident L15 L17.end
  measures "d167" distance of L13 L15
  measures "d168" distance of L12.end L18.end
extrude "Extrude43" add sketch "Sketch43" along normal blind 6.35 contours L0 L1 L13 L14 L15 L18 bodies 7
sketch "Sketch44" plane through (-6.35, 0, 0) normal (1, 0, 0) x (0, 1, 0)
  line L0 (292.1, 0) -> (304.8, 0)
  line L1 (304.8, 0) -> (304.8, 25.4)
  line L2 (304.8, 25.4) -> (311.15, 25.4)
  line L3 (311.15, 25.4) -> (311.15, 31.75)
  line L4 (311.15, 31.75) -> (304.8, 31.75)
  line L5 (304.8, 31.75) -> (304.8, 882.65)
  line L6 (304.8, 882.65) -> (311.15, 882.65)
  line L7 (311.15, 882.65) -> (311.15, 889)
  line L8 (311.15, 889) -> (304.8, 889)
  line L9 (304.8, 889) -> (304.8, 914.4)
  line L10 (304.8, 914.4) -> (292.1, 914.4)
  line L11 (292.1, 914.4) -> (292.1, 0)
  line L12 (292.1, 914.4) -> (298.45, 914.4)
  line L13 (298.45, 914.4) -> (298.45, 0)
  line L14 (298.45, 0) -> (292.1, 0)
  line L15 (292.1, 0) -> (292.1, 914.4)
  line L16 (292.1, 914.4) -> (298.45, 914.4)
  line L17 (298.45, 914.4) -> (298.45, 908.05)
  line L18 (298.45, 908.05) -> (292.1, 908.05)
  line L19 (292.1, 908.05) -> (292.1, 914.4)
  dimension "d171" = 6.35
  dimension "d172" = 6.35
  constraint horizontal L12
  constraint vertical L13
  constraint horizontal L14
  constraint vertical L15
  constraint coincident L0 L13.end
  constraint coincident L10.end L11.start
  constraint horizontal L16
  constraint vertical L17
  constraint horizontal L18
  constraint vertical L19
  constraint coincident L13 L17.end
  measures "d171" distance of L13 L15
  measures "d172" distance of L16 L18
extrude "Extrude44" add sketch "Sketch44" along normal blind 6.35 contours L0 L11 L13 L14 L15 L18 bodies 7
sketch "Sketch45" plane through (0, 0, 0) normal (0, 0, 1) x (1, 0, 0)
  line L0 (-63.8367, 309.571) -> (133.0133, 309.571)
  line L1 (133.0133, 309.571) -> (133.0133, 119.071)
  line L2 (133.0133, 119.071) -> (-63.8367, 119.071)
  line L3 (-63.8367, 119.071) -> (-63.8367, 309.571)
  line L4 (133.0133, 296.871) -> (-51.1367, 296.871)
  line L5 (-51.1367, 296.871) -> (-51.1367, 131.771)
  line L6 (-51.1367, 131.771) -> (133.0133, 131.771)
  line L7 (133.0133, 131.771) -> (133.0133, 296.871)
  dimension "d175" = 196.85
  dimension "d176" = 190.5
  dimension "d177" = 12.7
  dimension "d178" = 12.7
  dimension "d179" = 12.7
  constraint horizontal L0
  constraint vertical L1
  constraint horizontal L2
  constraint vertical L3
  constraint horizontal L4
  constraint vertical L5
  constraint horizontal L6
  constraint vertical L7
  constraint coincident L1 L4.start
  measures "d175" distance of L0.start L0.end
  measures "d176" distance of L0.start L2.end
  measures "d177" distance of L0 L4
  measures "d178" distance of L3 L5
  measures "d179" distance of L2 L6
extrude "Extrude45" add sketch "Sketch45" along normal blind 914.4 separate body contours L0 L1 L2 L3 L4 L5 L6 makes body 8
move_body "Move15" bodies 8 to x (-1, 0, 0) y (0, -1, 0) z (0, 0, 1) at (-102.2734, 475.1711, 0)
sketch "Sketch46" plane through (-235.2867, 0, 0) normal (-1, 0, 0) x (0, -1, 0)
  line L0 (-356.1002, 0) -> (-343.4002, 0)
  line L1 (-343.4002, 0) -> (-343.4002, 914.4)
  line L2 (-343.4002, 914.4) -> (-356.1002, 914.4)
  line L3 (-356.1002, 914.4) -> (-356.1002, 0)
  line L4 (-343.4002, 0) -> (-349.7502, 0)
  line L5 (-349.7502, 0) -> (-349.7502, 152.4)
  line L6 (-349.7502, 152.4) -> (-343.4002, 152.4)
  line L7 (-343.4002, 152.4) -> (-343.4002, 0)
  line L8 (-349.7502, 152.4) -> (-343.4002, 152.4)
  line L9 (-343.4002, 152.4) -> (-343.4002, 146.05)
  line L10 (-343.4002, 146.05) -> (-349.7502, 146.05)
  line L11 (-349.7502, 146.05) -> (-349.7502, 152.4)
  dimension "d182" = 6.35
  dimension "d183" = 6.35
  constraint horizontal L4
  constraint vertical L5
  constraint horizontal L6
  constraint vertical L7
  constraint coincident L0.end L1.start
  constraint horizontal L8
  constraint vertical L9
  constraint horizontal L10
  constraint vertical L11
  constraint coincident L7 L9.end
  measures "d182" distance of L0.end L4.end
  measures "d183" distance of L8 L10
extrude "Extrude46" cut sketch "Sketch46" against normal blind 6.35 contours L0 L1 L4 L5 L7 L10 bodies 8
sketch "Sketch47" plane through (-235.2867, 0, 0) normal (-1, 0, 0) x (0, -1, 0)
  line L0 (-178.3002, 0) -> (-165.6002, 0)
  line L1 (-165.6002, 0) -> (-165.6002, 914.4)
  line L2 (-165.6002, 914.4) -> (-178.3002, 914.4)
  line L3 (-178.3002, 914.4) -> (-178.3002, 0)
  line L4 (-178.3002, 0) -> (-171.9502, 0)
  line L5 (-171.9502, 0) -> (-171.9502, 152.4)
  line L6 (-171.9502, 152.4) -> (-178.3002, 152.4)
  line L7 (-178.3002, 152.4) -> (-178.3002, 0)
  line L8 (-178.3002, 152.4) -> (-171.9502, 152.4)
  line L9 (-171.9502, 152.4) -> (-171.9502, 146.05)
  line L10 (-171.9502, 146.05) -> (-178.3002, 146.05)
  line L11 (-178.3002, 146.05) -> (-178.3002, 152.4)
  dimension "d186" = 6.35
  dimension "d187" = 6.35
  constraint horizontal L4
  constraint vertical L5
  constraint horizontal L6
  constraint vertical L7
  constraint coincident L0.start L3.end
  constraint horizontal L8
  constraint vertical L9
  constraint horizontal L10
  constraint vertical L11
  constraint coincident L5 L9.end
  measures "d186" distance of L0.start L4.end
  measures "d187" distance of L8 L10
extrude "Extrude47" cut sketch "Sketch47" against normal blind 6.35 contours L0 L3 L4 L5 L7 L10 bodies 8
sketch "Sketch48" plane through (0, 356.1002, 0) normal (0, 1, 0) x (-1, 0, 0)
  line L0 (38.4367, 0) -> (235.2867, 0)
  line L1 (235.2867, 0) -> (235.2867, 914.4)
  line L2 (235.2867, 914.4) -> (38.4367, 914.4)
  line L3 (38.4367, 914.4) -> (38.4367, 0)
  line L4 (38.4367, 889) -> (235.2867, 889)
  line L5 (235.2867, 889) -> (235.2867, 882.65)
  line L6 (235.2867, 882.65) -> (38.4367, 882.65)
  line L7 (38.4367, 882.65) -> (38.4367, 889)
  dimension "d190" = 6.35
  dimension "d191" = 25.4
  constraint horizontal L4
  constraint vertical L5
  constraint horizontal L6
  constraint vertical L7
  constraint coincident L1 L5.end
  constraint coincident L3 L4.start
  measures "d190" distance of L4.start L6.end
  measures "d191" distance of L2 L4
extrude "Extrude48" add sketch "Sketch48" along normal blind 6.35 contours L1 L3 L4 L5 L6 L7 bodies 8
sketch "Sketch49" plane through (0, 356.1002, 0) normal (0, 1, 0) x (-1, 0, 0)
  line L0 (235.2867, 882.65) -> (38.4367, 882.65)
  line L1 (38.4367, 882.65) -> (38.4367, 0)
  line L2 (38.4367, 0) -> (235.2867, 0)
  line L3 (235.2867, 0) -> (235.2867, 882.65)
  line L4 (38.4367, 25.4) -> (235.2867, 25.4)
  line L5 (235.2867, 25.4) -> (235.2867, 31.75)
  line L6 (235.2867, 31.75) -> (38.4367, 31.75)
  line L7 (38.4367, 31.75) -> (38.4367, 25.4)
  dimension "d194" = 25.4
  dimension "d195" = 6.35
  constraint horizontal L4
  constraint vertical L5
  constraint horizontal L6
  constraint vertical L7
  constraint coincident L3 L5.end
  constraint coincident L1 L4.start
  measures "d194" distance of L2 L4
  measures "d195" distance of L4 L6
extrude "Extrude49" add sketch "Sketch49" along normal blind 6.35 contours L1 L3 L4 L5 L6 L7 bodies 8
sketch "Sketch50" plane through (0, 165.6002, 0) normal (0, -1, 0) x (1, 0, 0)
  line L0 (-235.2867, 0) -> (-38.4367, 0)
  line L1 (-38.4367, 0) -> (-38.4367, 914.4)
  line L2 (-38.4367, 914.4) -> (-235.2867, 914.4)
  line L3 (-235.2867, 914.4) -> (-235.2867, 0)
  line L4 (-235.2867, 882.65) -> (-38.4367, 882.65)
  line L5 (-38.4367, 882.65) -> (-38.4367, 889)
  line L6 (-38.4367, 889) -> (-235.2867, 889)
  line L7 (-235.2867, 889) -> (-235.2867, 882.65)
  dimension "d198" = 6.35
  dimension "d199" = 25.4
  constraint horizontal L4
  constraint vertical L5
  constraint horizontal L6
  constraint vertical L7
  constraint coincident L1 L5.end
  constraint coincident L3 L4.start
  measures "d198" distance of L4.start L6.end
  measures "d199" distance of L2 L6
extrude "Extrude50" add sketch "Sketch50" along normal blind 6.35 contours L1 L3 L4 L5 L6 L7 bodies 8
sketch "Sketch51" plane through (0, 165.6002, 0) normal (0, -1, 0) x (1, 0, 0)
  line L0 (-38.4367, 882.65) -> (-235.2867, 882.65)
  line L1 (-235.2867, 882.65) -> (-235.2867, 0)
  line L2 (-235.2867, 0) -> (-38.4367, 0)
  line L3 (-38.4367, 0) -> (-38.4367, 882.65)
  line L4 (-235.2867, 31.75) -> (-38.4367, 31.75)
  line L5 (-38.4367, 31.75) -> (-38.4367, 25.4)
  line L6 (-38.4367, 25.4) -> (-235.2867, 25.4)
  line L7 (-235.2867, 25.4) -> (-235.2867, 31.75)
  dimension "d202" = 25.4
  dimension "d203" = 6.35
  constraint horizontal L4
  constraint vertical L5
  constraint horizontal L6
  constraint vertical L7
  constraint coincident L3 L5.end
  constraint coincident L1 L4.start
  measures "d202" distance of L2 L6
  measures "d203" distance of L4 L6
extrude "Extrude51" add sketch "Sketch51" along normal blind 6.35 contours L1 L3 L4 L5 L6 L7 bodies 8
sketch "Sketch52" plane through (-38.4367, 0, 0) normal (1, 0, 0) x (0, 1, 0)
  line L0 (165.6002, 0) -> (356.1002, 0)
  line L1 (356.1002, 0) -> (356.1002, 25.4)
  line L2 (356.1002, 25.4) -> (362.4502, 25.4)
  line L3 (362.4502, 25.4) -> (362.4502, 31.75)
  line L4 (362.4502, 31.75) -> (356.1002, 31.75)
  line L5 (356.1002, 31.75) -> (356.1002, 882.65)
  line L6 (356.1002, 882.65) -> (362.4502, 882.65)
  line L7 (362.4502, 882.65) -> (362.4502, 889)
  line L8 (362.4502, 889) -> (356.1002, 889)
  line L9 (356.1002, 889) -> (356.1002, 914.4)
  line L10 (356.1002, 914.4) -> (165.6002, 914.4)
  line L11 (165.6002, 914.4) -> (165.6002, 889)
  line L12 (165.6002, 889) -> (159.2502, 889)
  line L13 (159.2502, 889) -> (159.2502, 882.65)
  line L14 (159.2502, 882.65) -> (165.6002, 882.65)
  line L15 (165.6002, 882.65) -> (165.6002, 31.75)
  line L16 (165.6002, 31.75) -> (159.2502, 31.75)
  line L17 (159.2502, 31.75) -> (159.2502, 25.4)
  line L18 (159.2502, 25.4) -> (165.6002, 25.4)
  line L19 (165.6002, 25.4) -> (165.6002, 0)
  line L20 (159.2502, 889) -> (362.4502, 889)
  line L21 (362.4502, 889) -> (362.4502, 882.65)
  line L22 (362.4502, 882.65) -> (159.2502, 882.65)
  line L23 (159.2502, 882.65) -> (159.2502, 889)
  constraint horizontal L20
  constraint vertical L21
  constraint horizontal L22
  constraint vertical L23
  constraint coincident L6.end L7.start
  constraint coincident L12.end L13.start
extrude "Extrude52" add sketch "Sketch52" along normal blind 6.35 contours L6 L7 L8 L12 L13 L14 L20 L21 L22 L23 bodies 8
sketch "Sketch53" plane through (-38.4367, 0, 0) normal (1, 0, 0) x (0, 1, 0)
  line L0 (356.1002, 882.65) -> (165.6002, 882.65)
  line L1 (165.6002, 882.65) -> (165.6002, 31.75)
  line L2 (165.6002, 31.75) -> (159.2502, 31.75)
  line L3 (159.2502, 31.75) -> (159.2502, 25.4)
  line L4 (159.2502, 25.4) -> (165.6002, 25.4)
  line L5 (165.6002, 25.4) -> (165.6002, 0)
  line L6 (165.6002, 0) -> (356.1002, 0)
  line L7 (356.1002, 0) -> (356.1002, 25.4)
  line L8 (356.1002, 25.4) -> (362.4502, 25.4)
  line L9 (362.4502, 25.4) -> (362.4502, 31.75)
  line L10 (362.4502, 31.75) -> (356.1002, 31.75)
  line L11 (356.1002, 31.75) -> (356.1002, 882.65)
  line L12 (159.2502, 31.75) -> (362.4502, 31.75)
  line L13 (362.4502, 31.75) -> (362.4502, 25.4)
  line L14 (362.4502, 25.4) -> (159.2502, 25.4)
  line L15 (159.2502, 25.4) -> (159.2502, 31.75)
  constraint horizontal L12
  constraint vertical L13
  constraint horizontal L14
  constraint vertical L15
  constraint coincident L8.end L9.start
  constraint coincident L2.end L3.start
extrude "Extrude53" add sketch "Sketch53" along normal blind 6.35 contours L2 L3 L4 L8 L9 L10 L12 L13 L14 L15 bodies 8
move_body "Move16" bodies 8 to x (1, 0, 0) y (0, 1, 0) z (0, 0, 1) at (0, -355.6, 190.5)
move_body "Move17" bodies 8 to x (1, 0, 0) y (0, 1, 0) z (0, 0, 1) at (0, 355.6, -152.4)
move_body "Move18" bodies 8 to x (1, 0, 0) y (0, 1, 0) z (0, 0, 1) at (0, 0, -50.8)
move_body "Move19" bodies 7 to x (1, 0, 0) y (0, 1, 0) z (0, 0, 1) at (-177.8, -342.9, 139.7)
move_body "Move20" bodies 7 to x (1, 0, 0) y (0, 1, 0) z (0, 0, 1) at (0, 6.35, 0)
move_body "Move21" bodies 7 to x (1, 0, 0) y (0, 1, 0) z (0, 0, 1) at (0, 0, -6.35)
move_body "Move22" bodies 7 to x (1, 0, 0) y (0, 1, 0) z (0, 0, 1) at (-6.35, 0, 0)
move_body "Move23" bodies 7 to x (1, 0, 0) y (0, 1, 0) z (0, 0, 1) at (50.8, 0, 0)
move_body "Move24" bodies 7 to x (1, 0, 0) y (0, 1, 0) z (0, 0, 1) at (0, 0, 50.8)
move_body "Move25" bodies 7 to x (1, 0, 0) y (0, 1, 0) z (0, 0, 1) at (0, 0, 25.4)
move_body "Move26" bodies 3 to x (1, 0, 0) y (0, 1, 0) z (0, 0, 1) at (0, 25.4, 0)
move_body "Move27" bodies 7 to x (1, 0, 0) y (0, 1, 0) z (0, 0, 1) at (0, 0, 406.4)
move_body "Move28" bodies 3 to x (1, 0, 0) y (0, 1, 0) z (0, 0, 1) at (0, 0, 50.8)
move_body "Move29" bodies 2 to x (1, 0, 0) y (0, 1, 0) z (0, 0, 1) at (63.5, 0, 0)
move_body "Move30" bodies 7 to x (1, 0, 0) y (0, 1, 0) z (0, 0, 1) at (76.2, -101.6, -431.8)
hidden bodies 6 8
equation "BaseX = 20 in" comment "The x axis of the Base"
equation "BaseY = 20 in" comment "The y axis of the Base"
equation "BaseZ = 8 in" comment "The z axis of the Base"
equation "TowerX = 8 in" comment "The x axis of the Tower"
equation "TowerY = 8 in" comment "The Y axis of the Tower"
equation "TowerZ = 36 in" comment "The z axis of the Tower"
equation "BaseThickness = 1 in" comment "The thickness of the base"
equation "TowerThickness = 0.5 in" comment "the thickness of the tower"
equation "d9 = BaseX"
equation "d10 = BaseY"
equation "d11 = BaseZ"
equation "d13 = BaseThickness"
equation "d14 = BaseThickness"
equation "d15 = BaseThickness"
equation "BaseCutOut = -( BaseZ - 1 in )" comment "How deep the box opens"
equation "d17 = BaseCutOut"
equation "BaseRabbit = BaseThickness / 2" comment "The length of the extruding fit"
equation "d20 = BaseRabbit"
equation "d21 = BaseRabbit"
equation "d22 = BaseRabbit"
equation "BaseDrop = 0.25 in" comment "The depth of the extruding fit"
equation "d24 = BaseDrop"
equation "d26 = BaseX"
equation "d27 = BaseY"
equation "d28 = BaseZ"
equation "d30 = BaseThickness"
equation "d31 = BaseThickness"
equation "d32 = BaseThickness"
equation "d33 = BaseCutOut"
equation "d35 = BaseRabbit"
equation "d36 = BaseRabbit"
equation "d37 = BaseRabbit"
equation "d38 = -BaseDrop"
equation "d40 = BaseX"
equation "d41 = BaseY"